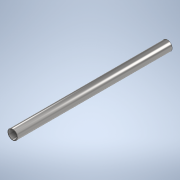
# Autodesk Inventor part: Barra_1_1-8_450
Saved by Autodesk Inventor 2021 (Build 250183000, 183)
## iProperties
Created: 2021-06-02
Part Number: Barra_1_1-8_450
Material: Steel, Mild
Document SubType Name: Modeling
Designer: Nelson
Density: 7.85 g/cm^3
Appearance: Semi-Polished
Mass: 450.704 g
Surface Area: 768.079 cm^2
Volume: 57.4146 cm^3
Author: Nelson
Autodesk Inventor part; units mm, degrees
ref_plane "YZ Plane" through (0, 0, 0) normal (1, 0, 0) x (0, 1, 0)
ref_plane "XZ Plane" through (0, 0, 0) normal (0, 1, 0) x (-1, 0, 0)
ref_plane "XY Plane" through (0, 0, 0) normal (0, 0, 1) x (1, 0, 0)
sketch "Sketch1" plane through (0, 0, 0) normal (0, 0, 1) x (1, 0, 0)
  circle A0 centre (0, 0) radius 14.2875
  circle A1 centre (0, 0) radius 12.7875
  dimension "d0" = 28.575
  dimension "d4" = 1.5
  constraints: 2 centre point, 2 coincident
  measures "d0" diameter of A0
  measures "d4" radial gap between concentric circles of A1 A0
extrude "Extrusion1" add sketch "Sketch1" against normal blind 450
body "Solid1"
